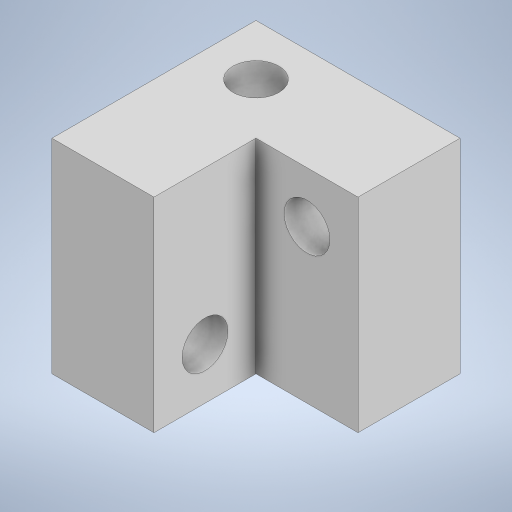
# Autodesk Inventor part: 부품81
Saved by Autodesk Inventor 2024 (Build 280153000, 153)
## iProperties
Created: 2024-09-09
Part Number: 부품81
Material: 일반
Document SubType Name: Modeling
Designer: Eungang
Density: 1 g/cm^3
Appearance: 기본값
Author: Eungang
Autodesk Inventor part; units mm, degrees
ref_plane "YZ Plane" through (0, 0, 0) normal (1, 0, 0) x (0, 1, 0)
ref_plane "XZ Plane" through (0, 0, 0) normal (0, 1, 0) x (-1, 0, 0)
ref_plane "XY Plane" through (0, 0, 0) normal (0, 0, 1) x (1, 0, 0)
sketch "스케치1" plane through (0, 0, 0) normal (0, 0, 1) x (1, 0, 0)
  line L0 (0, 0) -> (12, 0)
  line L1 (12, 0) -> (12, 12)
  line L2 (12, 12) -> (0, 12)
  line L3 (0, 12) -> (0, 0)
  dimension "d0" = 12
  dimension "d1" = 12
  constraints: 8 end point, 2 parallel, 1 horizontal, 1 perpendicular
  measures "d0" distance of L2.end L1.end
  measures "d1" distance of L1.end L0.end
extrude "돌출1" add sketch "스케치1" along normal blind 6
sketch "스케치2" plane through (0, 0, 6) normal (0, 0, 1) x (1, 0, 0)
  line L0 (12, 12) -> (0, 12) projected
  line L1 (0, 0) -> (6, 0)
  line L2 (6, 0) -> (6, 12)
  line L3 (6, 12) -> (0, 12)
  line L4 (0, 12) -> (0, 0)
  constraints: 8 end point, 2 parallel, 1 horizontal, 1 midpoint, 1 perpendicular
extrude "돌출2" add sketch "스케치2" along normal blind 6
sketch "스케치3" plane through (0, 0, 0) normal (0, -1, 0) x (1, 0, 0)
  line L0 (12, 6) -> (6, 6) projected
  line L1 (6, 6) -> (0, 6)
  line L2 (0, 6) -> (0, 0)
  line L3 (0, 0) -> (6, 0)
  line L4 (6, 0) -> (6, 6)
  circle A0 centre (3, 3) radius 1.35
  dimension "d6" = 2.7
  constraints: 8 end point, 2 parallel, 1 centre point, 1 horizontal, 1 perpendicular
  measures "d6" diameter of A0
extrude "돌출3" cut sketch "스케치3" against normal up to next contours A0
sketch "스케치4" plane through (0, 0, 0) normal (-1, 0, 0) x (0, 0, 1)
  line L0 (0, 0) -> (12, 0) projected
  line L1 (12, 0) -> (6, 0)
  line L2 (6, 0) -> (6, 6)
  line L3 (6, 6) -> (12, 6)
  line L4 (12, 6) -> (12, 0)
  circle A0 centre (9, 3) radius 1.35
  dimension "d9" = 2.7
  constraints: 8 end point, 2 parallel, 1 centre point, 1 horizontal, 1 perpendicular
  measures "d9" diameter of A0
extrude "돌출4" cut sketch "스케치4" against normal up to next contours A0
sketch "스케치5" plane through (0, 0, 6) normal (0, 0, 1) x (1, 0, 0)
  line L0 (12, 0) -> (12, 12) projected
  line L1 (12, 12) -> (6, 12)
  line L2 (6, 12) -> (6, 6)
  line L3 (6, 6) -> (12, 6)
  line L4 (12, 6) -> (12, 12)
  circle A0 centre (9, 9) radius 1.35
  point P0 (0, 0)
  dimension "d12" = 2.7
  constraints: 8 end point, 2 parallel, 1 centre point, 1 horizontal, 1 perpendicular
  measures "d12" diameter of A0
extrude "돌출5" cut sketch "스케치5" against normal up to next contours A0
